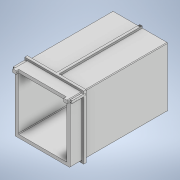
# Autodesk Inventor part: tacho
Saved by Autodesk Inventor 2021 (Build 250183000, 183)
## iProperties
Created: 2022-02-10
Part Number: tacho
Material: Genérico
Document SubType Name: Modeling
Designer: Emanuel
Density: 1 g/cm^3
Appearance: Valor por defecto
Author: Emanuel
Autodesk Inventor part; units mm, degrees
ref_plane "YZ Plane" through (0, 0, 0) normal (1, 0, 0) x (0, 1, 0)
ref_plane "XZ Plane" through (0, 0, 0) normal (0, 1, 0) x (-1, 0, 0)
ref_plane "XY Plane" through (0, 0, 0) normal (0, 0, 1) x (1, 0, 0)
sketch "Boceto1" plane through (0, 0, 0) normal (0, 0, 1) x (1, 0, 0)
  line L0 (-187.5, 210) -> (187.5, 210)
  line L1 (192.5, 205) -> (192.5, -205)
  line L2 (187.5, -210) -> (-187.5, -210)
  line L3 (-192.5, -205) -> (-192.5, 205)
  line L4 (-192.5, 210) -> (192.5, -210) construction
  line L5 (192.5, 210) -> (-192.5, -210) construction
  line L6 (-212.5, 235) -> (212.5, 235)
  line L7 (217.5, 230) -> (217.5, -230)
  line L8 (212.5, -235) -> (-212.5, -235)
  line L9 (-217.5, -230) -> (-217.5, 230)
  line L10 (-217.5, 235) -> (217.5, -235) construction
  line L11 (217.5, 235) -> (-217.5, -235) construction
  arc A0 (-212.5, 235) -> (-217.5, 230) centre (-212.5, 230) ccw
  arc A1 (-217.5, -230) -> (-212.5, -235) centre (-212.5, -230) ccw
  arc A2 (-192.5, -205) -> (-187.5, -210) centre (-187.5, -205) ccw
  arc A3 (187.5, -210) -> (192.5, -205) centre (187.5, -205) ccw
  arc A4 (212.5, -235) -> (217.5, -230) centre (212.5, -230) ccw
  arc A5 (192.5, 205) -> (187.5, 210) centre (187.5, 205) ccw
  arc A6 (217.5, 230) -> (212.5, 235) centre (212.5, 230) ccw
  arc A7 (-187.5, 210) -> (-192.5, 205) centre (-187.5, 205) ccw
  point P0 (0, 0)
  dimension "d17" = 5
  dimension "d26" = 470
  dimension "d27" = 385
  dimension "d39" = 435
  constraints: 24 end point, 16 point on circle, 16 point on line, 16 tangent, 8 centre point, 7 equal radius, 4 midpoint, 4 parallel, 2 horizontal, 2 perpendicular
  measures "d17" radius of A0
  measures "d26" distance between parallel lines of L8 L6
  measures "d27" distance between parallel lines of L1 L3
  measures "d39" distance between parallel lines of L7 L9
extrude "Extrusión1" add sketch "Boceto1" along normal blind 50 contours L0 A5 L1 A3 L2 A2 L3 A7
extrude "Extrusión2" add sketch "Boceto1" along normal blind 770
sketch "Boceto2" plane through (0, 0, 770) normal (0, 0, 1) x (1, 0, 0)
  line L0 (-212.6875, 235) -> (-187.5, 235)
  line L1 (212.5, 235) -> (-212.5, 235) projected
  line L2 (-187.5, 235) -> (-187.5, 210)
  line L3 (-187.5, 210) -> (-217.6875, 210)
  line L4 (-217.6875, 210) -> (-217.6875, 230)
  line L5 (-217.5, 230) -> (-217.5, -230) projected
  arc A0 (-212.6875, 235) -> (-217.6875, 230) centre (-212.6875, 230) ccw
  line L6 (212.6875, 235) -> (187.5, 235)
  line L7 (187.5, 235) -> (187.5, 210)
  line L8 (187.5, 210) -> (217.6875, 210)
  line L9 (217.6875, 210) -> (217.6875, 230)
  arc A1 (217.6875, 230) -> (212.6875, 235) centre (212.6875, 230) ccw
  point P0 (0, 0)
  constraints: 16 end point, 4 point on circle, 2 centre point, 2 tangent, 2 vertical, 1 perpendicular, 1 point on line, 1 other
extrude "Extrusión3" add sketch "Boceto2" along normal blind 20
sketch "Boceto3" plane through (217.6875, 210, 770) normal (1, 0, 0) x (0, 0, -1)
  line L0 (720, 0) -> (0, 0) projected
  line L1 (-20, 20) -> (0, 20)
  circle A0 centre (-10, 10) radius 5
  point P0 (770, -210)
  constraints: 2 end point, 1 centre point
extrude "Extrusión4" cut sketch "Boceto3" against normal up to surface (435.375 mm away)
sketch "Boceto4" plane through (-212.5, -235, 0) normal (0, -1, 0) x (1, 0, 0)
  line L0 (162.5, 677.5723) -> (262.5, 677.5723)
  line L1 (262.5, 677.5723) -> (262.5, 607.5723)
  line L2 (262.5, 607.5723) -> (162.5, 607.5723)
  line L3 (162.5, 607.5723) -> (162.5, 677.5723)
  line L4 (169.5157, 652.5723) -> (212.5157, 652.5723)
  line L5 (212.5157, 652.5723) -> (212.5157, 632.5723)
  line L6 (212.5157, 632.5723) -> (169.5157, 632.5723)
  line L7 (169.5157, 632.5723) -> (169.5157, 652.5723)
  circle A0 centre (244.0773, 642.3979) radius 5
  circle A1 centre (244.0773, 662.3979) radius 5
  circle A2 centre (244.0773, 622.3979) radius 5
  point P0 (212.5, 0)
  point P1 (191.0157, 642.5723)
  constraints: 16 end point, 4 parallel, 3 centre point, 2 horizontal, 2 perpendicular
extrude "Extrusión5" add sketch "Boceto4" along normal blind 15
sketch "Boceto5" plane through (-212.5, -235, 0) normal (0, -1, 0) x (1, 0, 0)
  line L0 (262.5, 607.5723) -> (262.5, 677.5723) projected
  line L1 (430, 0) -> (430, 770) projected
  line L2 (262.5, 677.5723) -> (430, 677.5723)
  line L3 (430, 677.5723) -> (430, 657.5723)
  line L4 (430, 657.5723) -> (262.5, 657.5723)
  line L5 (262.5, 657.5723) -> (262.5, 677.5723)
  point P0 (212.5, 0)
  dimension "d40" = 20
  constraints: 8 end point, 2 parallel, 1 horizontal, 1 perpendicular, 1 point on line
  measures "d40" distance of L2.end L3.end
extrude "Extrusión6" add sketch "Boceto5" along normal blind 15
sketch "Boceto6" plane through (217.5, -230, 0) normal (1, 0, 0) x (0, 0, -1)
  line L0 (-677.5723, -5) -> (-677.5723, -20) projected
  line L1 (-677.5723, -20) -> (-657.5723, -20)
  line L2 (-657.5723, -20) -> (-657.5723, 465)
  line L3 (-657.5723, 465) -> (-677.5723, 465)
  line L4 (-677.5723, 465) -> (-677.5723, -20)
  line L5 (-50, 440) -> (-770, 440) projected
  line L6 (-770, 440) -> (-657.5723, 440)
  line L7 (-657.5723, 440) -> (-657.5723, 465)
  line L8 (-770, 440) -> (-770, 0) projected
  line L9 (-770, 465) -> (-770, 460) projected
  line L10 (-770, 440) -> (-770, 460)
  line L11 (-770, 460) -> (-677.5723, 460)
  line L12 (0, 460) -> (-770, 460) projected
  point P0 (0, 230)
  point P1 (-677.5723, 440)
  dimension "d43" = 20
  constraints: 16 end point, 2 horizontal, 2 parallel, 2 perpendicular, 2 point on line, 1 vertical
  measures "d43" distance of L3.end L2.end
extrude "Extrusión7" add sketch "Boceto6" along normal blind 15
sketch "Boceto8" plane through (-212.5, 235, 0) normal (0, 1, 0) x (1, 0, 0)
  line L0 (-5, 0) -> (-5, -770) projected
  line L1 (445, -657.5723) -> (-5, -657.5723)
  line L2 (-5, -657.5723) -> (-5, -677.5723)
  line L3 (-5, -677.5723) -> (445, -677.5723)
  line L4 (445, -677.5723) -> (445, -657.5723)
  line L5 (0, 0) -> (425, 0) projected
  line L6 (230.8697, -657.5723) -> (210.8697, -657.5723)
  line L7 (210.8697, -657.5723) -> (210.8697, 0)
  line L8 (210.8697, 0) -> (230.8697, 0)
  line L9 (230.8697, 0) -> (230.8697, -657.5723)
  point P0 (212.5, 0)
  dimension "d48" = 20
  dimension "d58" = 20
  constraints: 16 end point, 4 parallel, 3 point on line, 2 horizontal, 2 perpendicular
  measures "d48" distance of L2.end L1.end
  measures "d58" distance of L7.end L8.end
extrude "Extrusión9" add sketch "Boceto8" along normal blind 15
sketch "Boceto9" plane through (-217.5, -230, 0) normal (-1, 0, 0) x (0, 0, 1)
  line L0 (770, 460) -> (770, 465) projected
  line L1 (657.5723, -20) -> (657.5723, 480) projected
  line L2 (770, 460) -> (657.5723, 460)
  line L3 (657.5723, 460) -> (657.5723, 440)
  line L4 (657.5723, 440) -> (770, 440)
  line L5 (770, 440) -> (770, 460)
  line L6 (677.5723, 465) -> (677.5723, 480) projected
  line L7 (677.5723, 480) -> (657.5723, 480)
  line L8 (657.5723, 480) -> (657.5723, 440)
  line L9 (657.5723, 440) -> (677.5723, 440)
  line L10 (677.5723, 440) -> (677.5723, 480)
  point P0 (0, 230)
  point P1 (677.5723, 460)
  dimension "d51" = 20
  constraints: 16 end point, 4 parallel, 2 horizontal, 2 perpendicular, 1 point on line
  measures "d51" distance of L3.end L2.end
extrude "Extrusión10" add sketch "Boceto9" along normal blind 15
sketch "Boceto10" plane through (-232.5, 230, 770) normal (0, 0, 1) x (1, 0, 0)
  line L0 (13.4835, -17.4072) -> (1.6576, -17.4072)
  line L1 (1.6576, -17.4072) -> (1.6576, -2.7657)
  line L2 (1.6576, -2.7657) -> (13.4835, -2.7657)
  line L3 (13.4835, -2.7657) -> (13.4835, -17.4072)
  point P0 (232.5, -230)
  constraints: 8 end point, 2 parallel, 1 horizontal, 1 perpendicular
extrude "Extrusión11" cut sketch "Boceto10" against normal blind 110
sketch "Boceto11" plane through (217.6875, 210, 770) normal (0, 0, 1) x (1, 0, 0)
  line L0 (1.6316, 2.047) -> (13.3887, 2.047)
  line L1 (13.3887, 2.047) -> (13.3887, 18.3261)
  line L2 (13.3887, 18.3261) -> (1.6316, 18.3261)
  line L3 (1.6316, 18.3261) -> (1.6316, 2.047)
  point P0 (-217.6875, -210)
  constraints: 8 end point, 2 parallel, 1 horizontal, 1 perpendicular
extrude "Extrusión12" cut sketch "Boceto11" against normal blind 110
sketch "Boceto12" plane through (-212.5, 250, 0) normal (0, 1, 0) x (1, 0, 0)
  line L0 (226.9474, -15.5762) -> (213.9056, -15.5762)
  line L1 (213.9056, -15.5762) -> (213.9056, -3.0365)
  line L2 (213.9056, -3.0365) -> (226.9474, -3.0365)
  line L3 (226.9474, -3.0365) -> (226.9474, -15.5762)
  point P0 (212.5, 0)
  constraints: 8 end point, 2 parallel, 1 horizontal, 1 perpendicular
extrude "Extrusión13" cut sketch "Boceto12" against normal blind 13.25
